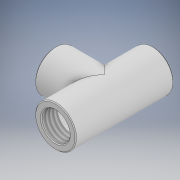
# Autodesk Inventor part: Verbindungsstück
Saved by Autodesk Inventor 2021 (Build 250183000, 183)
## iProperties
Created: 2021-11-19
Part Number: Verbindungsstück
Material: Generisch
Document SubType Name: Modeling
Designer: lukas
Density: 1 g/cm^3
Appearance: Vorgabe
Author: lukas
Autodesk Inventor part; units mm, degrees
ref_plane "YZ Plane" through (0, 0, 0) normal (1, 0, 0) x (0, 1, 0)
ref_plane "XZ Plane" through (0, 0, 0) normal (0, 1, 0) x (-1, 0, 0)
ref_plane "XY Plane" through (0, 0, 0) normal (0, 0, 1) x (1, 0, 0)
sketch "Skizze1" plane through (0, 0, 0) normal (0, 0, 1) x (1, 0, 0)
  line L0 (-17.5, 0) -> (17.5, 0) projected
  line L1 (0, -17.5) -> (0, 17.5) projected
  circle A0 centre (0, 0) radius 12.5
  dimension "d0" = 25
  constraints: 1 centre point, 1 coincident
  measures "d0" diameter of A0
extrude "Extrusion1" add sketch "Skizze1" along normal blind 60
sketch "Skizze2" plane through (0, 0, 60) normal (0, 0, 1) x (1, 0, 0)
  circle A0 centre (0, 0) radius 10.8915
  constraints: 1 centre point, 1 coincident
sketch "Skizze3" plane through (0, 0, 0) normal (1, 0, 0) x (0, 1, 0)
  line L0 (12.5, 0) -> (-12.5, 0) projected
  circle A0 centre (0, 30) radius 12.5
  point P0 (0, 0)
  dimension "d3" = 30
  dimension "d4" = 25
  constraints: 1 centre point, 1 coincident
  measures "d3" distance from line of point (0, 30) L0
  measures "d4" diameter of A0
extrude "Extrusion2" add sketch "Skizze3" against normal blind 30
sketch "Skizze4" plane through (0, 0, 0) normal (0, 0, -1) x (-1, 0, 0)
  point P0 (0, 0)
hole "Bohrung1" at (0, 0, 0) direction (0, 0, 1) diameter 17.294 depth 30 thread size "M20x2.5" class "6H" standard "ISO Metric profile"
hole "Bohrung2" at (0, 0, 60) direction (0, 0, -1) diameter 17.294 depth 30 thread size "M20x2.5" class "6H" standard "ISO Metric profile"
sketch "Skizze5" plane through (-30, 0, 30) normal (-1, 0, 0) x (0, 0, 1)
  point P0 (-30, 0)
  point P1 (0.0118, -0.0059)
hole "Bohrung3" at (-30, -0.0059, 30.0118) direction (1, 0, 0) diameter 17.294 depth 30 thread size "M20x2.5" class "6H" standard "ISO Metric profile"
chamfer "Fase1" distance 0.5 angle 45 6 edges at (-12.5, 0, 60) (0, 8.647, 60) (-30, -12.5, 30) (-30, -0.0059, 21.3648) (-12.5, 0, 0) (0, -8.647, 0)
